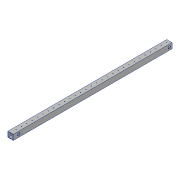
# Autodesk Inventor part: Support Pivs 25 upper
Saved by Autodesk Inventor 2018 (Build 220112000, 112)
## iProperties
Created: 2018-01-08
Part Number: Support Pivs 25 upper
Material: Aluminum 6061
Document SubType Name: Modeling
Designer: dsayers
Density: 2.7 g/cm^3
Appearance: Aluminum - Flat
Mass: 440.569 g
Surface Area: 1304.88 cm^2
Volume: 163.174 cm^3
Author: dsayers
Autodesk Inventor part; units mm, degrees
ref_plane "YZ Plane" through (0, 0, 0) normal (1, 0, 0) x (0, 1, 0)
ref_plane "XZ Plane" through (0, 0, 0) normal (0, 1, 0) x (-1, 0, 0)
ref_plane "XY Plane" through (0, 0, 0) normal (0, 0, 1) x (1, 0, 0)
sketch "Sketch1" plane through (0, 0, 0) normal (0, 0, 1) x (1, 0, 0)
  line L0 (0, 0) -> (25.4, 0)
  line L1 (25.4, 0) -> (25.4, 25.4)
  line L2 (25.4, 25.4) -> (0, 25.4)
  line L3 (0, 25.4) -> (0, 0)
  dimension "d0" = 25.4
  dimension "d1" = 25.4
  constraints: 8 end point, 2 parallel, 1 horizontal, 1 perpendicular
  measures "d0" distance of L1.end L2.end
  measures "d1" distance of L0.end L1.end
extrude "Extrusion1" add sketch "Sketch1" along normal blind 749.3
shell "Shell1" thickness 2.54 removed faces 2 at (8.4667, 16.9333, 0) at (8.4667, 16.9333, 749.3)
sketch "Sketch2" plane through (0, 25.4, 0) normal (0, 1, 0) x (1, 0, 0)
  line L0 (25.4, 0) -> (0, 0) projected
  line L1 (0, 0) -> (0, -749.3) projected
  point P0 (12.7, -12.7)
  point P1 (12.7, -38.1)
  point P2 (12.7, -63.5)
  point P3 (12.7, -88.9)
  point P4 (12.7, -114.3)
  point P5 (12.7, -139.7)
  point P6 (12.7, -165.1)
  point P7 (12.7, -190.5)
  point P8 (12.7, -215.9)
  point P9 (12.7, -241.3)
  point P10 (12.7, -266.7)
  point P11 (12.7, -292.1)
  point P12 (12.7, -317.5)
  point P13 (12.7, -342.9)
  point P14 (12.7, -368.3)
  point P15 (12.7, -393.7)
  point P16 (12.7, -419.1)
  point P17 (12.7, -444.5)
  point P18 (12.7, -469.9)
  point P19 (12.7, -495.3)
  point P20 (12.7, -520.7)
  point P21 (12.7, -546.1)
  point P22 (12.7, -571.5)
  point P23 (12.7, -596.9)
  point P24 (12.7, -622.3)
  point P25 (12.7, -647.7)
  point P26 (12.7, -673.1)
  point P27 (12.7, -698.5)
  point P28 (12.7, -723.9)
  point P29 (12.7, -749.3)
  point P30 (12.7, -774.7)
  point P31 (12.7, -800.1)
  point P32 (12.7, -825.5)
  point P33 (12.7, -850.9)
  point P34 (12.7, -876.3)
  point P35 (12.7, -901.7)
  point P36 (12.7, -927.1)
  dimension "d5" = 12.7
  dimension "d6" = 12.7
  dimension "d9" = 25.4
  constraints: 1 vertical, 36 other
  measures "d5" distance from line of L0 point (12.7, -12.7)
  measures "d6" distance from line of L1 point (12.7, -12.7)
  measures "d9" distance of point (12.7, -12.7) point (12.7, -38.1)
hole "Hole1" at (12.7, 25.4, 12.7) at (12.7, 25.4, 38.1) at (12.7, 25.4, 63.5) at (12.7, 25.4, 88.9) at (12.7, 25.4, 114.3) at (12.7, 25.4, 139.7) at (12.7, 25.4, 165.1) at (12.7, 25.4, 190.5) at (12.7, 25.4, 215.9) at (12.7, 25.4, 241.3) at (12.7, 25.4, 266.7) at (12.7, 25.4, 292.1) at (12.7, 25.4, 317.5) at (12.7, 25.4, 342.9) at (12.7, 25.4, 368.3) at (12.7, 25.4, 393.7) at (12.7, 25.4, 419.1) at (12.7, 25.4, 444.5) at (12.7, 25.4, 469.9) at (12.7, 25.4, 495.3) at (12.7, 25.4, 520.7) at (12.7, 25.4, 546.1) at (12.7, 25.4, 571.5) at (12.7, 25.4, 596.9) at (12.7, 25.4, 622.3) at (12.7, 25.4, 647.7) at (12.7, 25.4, 673.1) at (12.7, 25.4, 698.5) at (12.7, 25.4, 723.9) at (12.7, 25.4, 749.3) at (12.7, 25.4, 774.7) at (12.7, 25.4, 800.1) at (12.7, 25.4, 825.5) at (12.7, 25.4, 850.9) at (12.7, 25.4, 876.3) at (12.7, 25.4, 901.7) direction (0, -1, 0) diameter 2.54 depth 50.8 tip angle 118
sketch "Sketch8" plane through (25.4, 0, 0) normal (1, 0, 0) x (0, 0, -1)
  line L0 (-749.3, 0) -> (-749.3, 25.4) projected
  line L1 (0, 25.4) -> (-749.3, 25.4) projected
  line L2 (0, 0) -> (0, 25.4) projected
  point P0 (-12.7, 12.7)
  point P1 (-723.9, 12.7)
  dimension "d57" = 25.4
  dimension "d58" = 12.7
  dimension "d59" = 12.7
  dimension "d60" = 12.7
  measures "d57" distance from line of L0 point (-723.9, 12.7)
  measures "d58" distance from line of L1 point (-723.9, 12.7)
  measures "d59" distance from line of L2 point (-12.7, 12.7)
  measures "d60" distance from line of L1 point (-12.7, 12.7)
hole "Hole5" at (25.4, 12.7, 12.7) at (25.4, 12.7, 723.9) direction (-1, 0, 0) diameter 12.7 depth 25.4 tip angle 118
body "Solid1"
